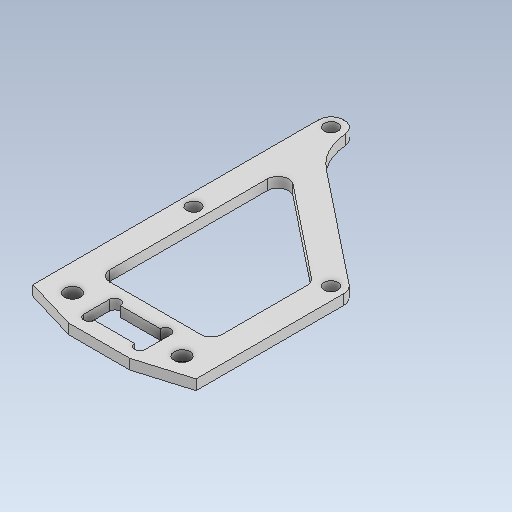
# Autodesk Inventor part: UpperArm_side_frame
Saved by Autodesk Inventor 2020.4 (Build 244396000, 396)
## iProperties
Created: 2021-09-30
Part Number: UpperArm_side_frame
Material: GFRP
Document SubType Name: Modeling
Designer: naoki
Density: 1.75 g/cm^3
Appearance: 滑らか - 淡い灰色
Description: GFRP T2
Mass: 2.60378 g
Surface Area: 21.8783 cm^2
Volume: 1.48787 cm^3
Author: Naoki Iwasawa
Autodesk Inventor part; units mm, degrees
ref_plane "YZ Plane" through (0, 0, 0) normal (1, 0, 0) x (0, 1, 0)
ref_plane "XZ Plane" through (0, 0, 0) normal (0, 1, 0) x (-1, 0, 0)
ref_plane "XY Plane" through (0, 0, 0) normal (0, 0, 1) x (1, 0, 0)
sketch "スケッチ1" plane through (0, 0, 0) normal (0, 1, 0) x (-1, 0, 0)
  line L0 (-16, 21.5) -> (16, 21.5) construction
  line L1 (16, 21.5) -> (16, -21.5) construction
  line L2 (16, -21.5) -> (-16, -21.5) construction
  line L3 (-16, -21.5) -> (-16, 21.5) construction
  line L4 (-16, 21.5) -> (16, -21.5) construction
  line L5 (16, 21.5) -> (-16, -21.5) construction
  line L6 (0, -35.1049) -> (0, 50.5) construction
  line L7 (34.5893, 0) -> (-34.3502, 0) construction
  circle A0 centre (0, -9.5) radius 10.5 construction
  arc A1 (-16, -9.5) -> (-10.5361, -21.5412) centre (0, -9.5) ccw construction
  arc A2 (10.5361, -21.5412) -> (16, -9.5) centre (0, -9.5) ccw construction
  circle A3 centre (-13.5, -8.5) radius 1.3 construction
  circle A4 centre (-13.5, 18.5) radius 1.3 construction
  circle A5 centre (13.5, -8.5) radius 1.3 construction
  circle A6 centre (13.5, 18.5) radius 1.3 construction
  line L8 (-16, 18.5) -> (-16, 50.5)
  line L9 (16, 18.5) -> (16, 50.5)
  line L10 (16, 50.5) -> (-16, 50.5) construction
  line L11 (6, 42.5) -> (0, 42.5) construction
  line L12 (16, 47.5) -> (6, 47.5) construction
  line L13 (-16, 47.5) -> (-6, 50.5)
  line L14 (6, 50.5) -> (-6, 50.5)
  circle A7 centre (-10.75, 45) radius 1.55
  circle A8 centre (10.75, 45) radius 1.55
  circle A9 centre (0, -9.5) radius 11
  line L15 (13.5, -8.5) -> (13.5, -8.5) construction
  line L16 (13.5, -7.15) -> (13.5, -7.15)
  line L17 (13.5, -9.85) -> (13.5, -9.85)
  arc A10 (13.5, -9.85) -> (13.5, -7.15) centre (13.5, -8.5) ccw
  arc A11 (13.5, -7.15) -> (13.5, -9.85) centre (13.5, -8.5) ccw
  line L18 (-13.5, -8.5) -> (-13.5, -8.5) construction
  line L19 (-13.5, -7.15) -> (-13.5, -7.15)
  line L20 (-13.5, -9.85) -> (-13.5, -9.85)
  arc A12 (-13.5, -7.15) -> (-13.5, -9.85) centre (-13.5, -8.5) ccw
  arc A13 (-13.5, -9.85) -> (-13.5, -7.15) centre (-13.5, -8.5) ccw
  arc A14 (-15.0569, 16.544) -> (-16, 18.5) centre (-13.5, 18.5) ccw construction
  arc A15 (-16, 18.5) -> (-15.0569, 16.544) centre (-13.5, 18.5) ccw
  line L21 (16, 18.5) -> (16, -8.5)
  arc A16 (13.5, -11) -> (16, -8.5) centre (13.5, -8.5) ccw
  circle A17 centre (-13.5, 18.5) radius 1.35
  circle A18 centre (13.5, 18.5) radius 1.35
  line L22 (-15.0569, 16.544) -> (6.8505, -0.8935)
  line L23 (16, 42.5) -> (6, 42.5) construction
  line L24 (11, 39.5) -> (-11, 39.5)
  line L25 (11, 2.1941) -> (11, 39.5)
  line L26 (11, 2.1941) -> (-11, 19.7054)
  line L27 (-11, 19.7054) -> (-11, 39.5)
  line L28 (6, 42.5) -> (-6, 42.5) construction
  line L29 (6, 47.5) -> (-16, 47.5) construction
  line L30 (-6, 42.5) -> (-16, 42.5) construction
  line L31 (-6, 47.5) -> (6, 47.5) construction
  line L32 (6, 47.5) -> (6, 42.5) construction
  line L33 (6, 42.5) -> (-6, 42.5) construction
  line L34 (-6, 42.5) -> (-6, 47.5) construction
  line L35 (-6, 47.5) -> (6, 42.5) construction
  line L36 (6, 47.5) -> (-6, 42.5) construction
  line L37 (16, 47.5) -> (6, 50.5)
  line L38 (6, 42.5) -> (-6, 42.5) construction
  line L39 (-6, 42.5) -> (-6, 47.5) construction
  line L40 (-6, 47.5) -> (6, 47.5) construction
  line L41 (6, 47.5) -> (6, 42.5) construction
  line L42 (6.01, 42.49) -> (-6.01, 42.49)
  line L43 (-6.01, 42.49) -> (-6.01, 47.51)
  line L44 (-6.01, 47.51) -> (6.01, 47.51)
  line L45 (6.01, 47.51) -> (6.01, 42.49)
  line L46 (6.01, 45) -> (-6.01, 45) construction
  arc A19 (-6.01, 42.49) -> (-3.91, 42.5) centre (-4.96, 42.49) ccw
  line L47 (0, 125.1049) -> (0, 39.5) construction
  arc A20 (-3.91, 47.5) -> (-6.01, 47.51) centre (-4.96, 47.51) ccw
  arc A21 (3.91, 42.5) -> (6.01, 42.49) centre (4.96, 42.49) ccw
  arc A22 (6.01, 47.51) -> (3.91, 47.5) centre (4.96, 47.51) ccw
  line L48 (13.5, -11) -> (10.8972, -11)
  point P0 (0, 0)
  point P1 (0, 0)
  point P2 (0, 0)
  point P3 (13.5, -8.5)
  point P4 (-13.5, -8.5)
  point P5 (0, 45)
  point P6 (0, 45)
  point P7 (3.91, 42.49)
  point P8 (-3.91, 42.49)
  point P9 (-3.91, 47.51)
  point P10 (3.91, 47.51)
  dimension "d0" = 32
  dimension "d1" = 43
  dimension "d2" = 9.5
  dimension "d3" = 8.5
  dimension "d4" = 18.5
  dimension "d5" = 13.5
  dimension "d6" = 13.5
  dimension "d7" = 21
  dimension "d8" = 16
  dimension "d9" = 2.6
  dimension "d10" = 2.6
  dimension "d17" = 32
  dimension "d18" = 32
  dimension "d26" = 3.1
  dimension "d30" = 22
  dimension "d31" = 2.7
  dimension "d32" = 3
  dimension "d33" = 5
  dimension "d34" = 5
  dimension "d35" = 5
  dimension "d36" = 3
  dimension "d37" = 5
  dimension "d38" = 10
  dimension "d39" = 10
  dimension "d40" = 3
  dimension "d41" = 10
  dimension "d42" = 0.01
  dimension "d43" = 1.05
  dimension "d48" = 21.5
  dimension "d49" = 1.35
  dimension "d51" = 0
  constraints: 102 end point, 28 point on circle, 25 symmetric about line, 23 centre point, 20 point on line, 13 parallel, 12 midpoint, 11 perpendicular, 10 coincident, 8 tangent, 7 horizontal, 2 collinear, 2 horizontal alignment, 1 vertical, 13 other
  measures "d0" distance of L1.end L2.end
  measures "d1" distance of L0.end L1.end
  measures "d2" distance of point (0, 0) point (0, -9.5)
  measures "d3" distance from line of point (-13.5, -8.5) L7
  measures "d4" distance from line of L7 point (-13.5, 18.5)
  measures "d5" distance from line of L6 point (-13.5, -8.5)
  measures "d6" distance from line of L6 point (-13.5, 18.5)
  measures "d7" diameter of A0
  measures "d8" radius of A1
  measures "d9" diameter of A3
  measures "d10" diameter of A4
  measures "d17" distance of L8.start L8.end
  measures "d18" distance of L9.start L9.end
  measures "d26" diameter of A7
  measures "d30" diameter of A9
  measures "d31" diameter of A17
  measures "d32" distance between parallel lines of L23 L24
  measures "d33" distance between parallel lines of L22 L26
  measures "d34" distance between parallel lines of L8 L27
  measures "d35" distance between parallel lines of L25 L9
  measures "d36" distance between parallel lines of L14 L31
  measures "d37" distance of L33.end L31.start
  measures "d38" distance between parallel lines of L8 L34
  measures "d39" distance from line of L8 L13.end
  measures "d40" distance from line of L10 L13.start
  measures "d41" distance from line of L9 L14.start
  measures "d42" distance between parallel lines of L33 L42
  measures "d43" distance from line of L43 point (-4.96, 42.49)
  measures "d48" distance of A7.centre A8.centre
  measures "d49" radius of A12
  measures "d51" distance of L18.end A3.centre
extrude "押し出し1" add sketch "スケッチ1" along normal blind 2 contours L8 L13 L14 L37 L9 L21 A16 L48 A9 L22 A15
fillet "フィレット1" radius 2.1 4 edges at (-11, 1, 2.1941) (11, 1, 39.5) (-11, 1, 39.5) (11, 1, 19.7054)
fillet "フィレット2" radius 2.5 1 edges at (-10.8972, 1, -11)
equation "\"d6\" = d5"
equation "\"d18\" = d17"
